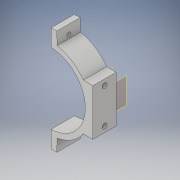
# Autodesk Inventor part: spannringe
Saved by Autodesk Inventor 2017 (Build 210142000, 142)
## iProperties
Part Number: spannringe
Material: Generisch
Document SubType Name: Modeling
Designer: Fabio
Density: 1 g/cm^3
Appearance: Vorgabe
Author: Fabio
Autodesk Inventor part; units mm, degrees
ref_plane "YZ Plane" through (0, 0, 0) normal (1, 0, 0) x (0, 1, 0)
ref_plane "XZ Plane" through (0, 0, 0) normal (0, 1, 0) x (-1, 0, 0)
ref_plane "XY Plane" through (0, 0, 0) normal (0, 0, 1) x (1, 0, 0)
sketch "Skizze1" plane through (0, 0, 0) normal (0, 1, 0) x (-1, 0, 0)
  arc A0 (-1, 30.4836) -> (-30.5, 0) centre (0, 0) ccw
  arc A1 (-6.2857, 34.431) -> (-35, 0) centre (0, 0) ccw
  line L0 (-1, 45) -> (-5.9982, 45.1342)
  line L1 (-5.9982, 45.1342) -> (-6.2857, 34.431)
  line L2 (0, 0) -> (-14.1914, 0) construction
  line L3 (-1, 30.4836) -> (-1, 45)
  arc A2 (-30.5, 0) -> (-1, -30.4836) centre (0, 0) ccw
  arc A3 (-35, 0) -> (-6.2857, -34.431) centre (0, 0) ccw
  line L4 (-1, -45) -> (-5.9982, -45.1342)
  line L5 (-5.9982, -45.1342) -> (-6.2857, -34.431)
  line L6 (-1, -30.4836) -> (-1, -45)
  dimension "d59" = 30.5
  dimension "d60" = 35
  dimension "d72" = 1
  dimension "d73" = 5
  dimension "d74" = 45
  dimension "d75" = 10.7071
  constraints: 14 end point, 9 coincident, 8 point on circle, 4 centre point, 4 symmetric about line, 1 horizontal, 1 perpendicular, 1 vertical, 2 other
  measures "d59" radius of A0
  measures "d60" radius of A1
  measures "d72" distance from line of point (0, 0) L3
  measures "d73" distance of L0.start L0.end
  measures "d74" vertical distance of point (0, 0) L0.start
  measures "d75" distance of L0.end L1.end
extrude "Extrusion1" add sketch "Skizze1" along normal blind 20
ref_plane "Arbeitsebene1" through (35, 20, 0) normal (1, 0, 0) x (0, 1, 0)
sketch "Skizze3" plane through (35, 20, 0) normal (1, 0, 0) x (0, 1, 0)
  line L0 (0, -30.4836) -> (0, 30.4836) projected
  line L1 (0, 20) -> (-20, 20)
  line L2 (-20, 20) -> (-20, -20)
  line L3 (-20, -20) -> (0, -20)
  line L4 (0, -20) -> (0, 20)
  point P0 (-20, 0)
  dimension "d28" = 20
  dimension "d30" = 20
  dimension "d31" = 20
  constraints: 8 end point, 2 parallel, 1 horizontal, 1 perpendicular, 1 point on line
  measures "d28" distance between parallel lines of L0 L2
  measures "d30" distance from line of L3 point (-20, 0)
  measures "d31" distance of L1.end point (-20, 0)
extrude "Extrusion2" add sketch "Skizze3" against normal blind 10 and the other way blind 2
sketch "Skizze5" plane through (1, 0, 30.4836) normal (-1, 0, 0) x (0, 0, 1)
  line L0 (14.5, 0) -> (14.5, 20) construction
  line L1 (14.5, 10) -> (-75.5, 10) construction
  line L2 (-75.5, 0) -> (-75.5, 20) construction
  line L3 (-75.5, 20) -> (-61, 20) construction
  line L4 (-68.25, 20) -> (-68.25, 0) construction
  line L5 (-61, 0) -> (-75.5, 0) construction
  line L6 (0, 20) -> (14.5, 20) construction
  line L7 (7.25, 20) -> (7.25, 0) construction
  line L8 (14.5, 0) -> (0, 0) construction
  point P0 (-30.5, 0)
  point P1 (7.25, 10)
  point P2 (-68.25, 10)
  constraints: 18 end point, 8 midpoint
hole "Bohrung3" at (1, 10, 37.7336) at (1, 10, -37.7664) direction (1, 0, 0) diameter 3.3 end through all
ref_plane "Arbeitsebene2" through (23, 20, 0) normal (1, 0, 0) x (0, 1, 0)
sketch "Skizze7" plane through (23, 20, 0) normal (1, 0, 0) x (0, 1, 0)
  line L0 (0, 30.4836) -> (0, -30.4836) projected
  point P0 (-20, 0)
  point P1 (-10, 15)
  point P2 (-10, -15)
  dimension "d81" = 10
  dimension "d82" = 10
  dimension "d84" = 15
  dimension "d94" = 15
  measures "d81" distance from line of L0 point (-10, 15)
  measures "d82" distance from line of L0 point (-10, -15)
  measures "d84" vertical distance of point (-20, 0) point (-10, 15)
  measures "d94" vertical distance of point (-10, -15) point (-20, 0)
hole "Bohrung4" at (23, 10, 15) at (23, 10, -15) direction (1, 0, 0) diameter 4.3 end through all counterbore diameter 8 counterbore depth 8
delete faces "Fläche löschen1" heal yes whole lump no faces at (25, 2.4288, 4.0204)
